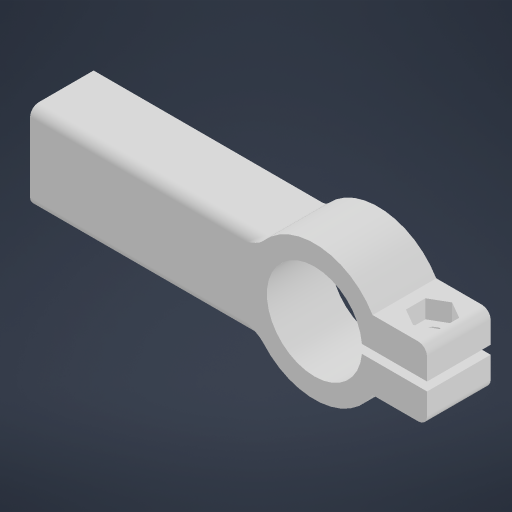
# Autodesk Inventor part: Clasp
Saved by Autodesk Inventor 2024.1 (Build 281209000, 209)
## iProperties
Created: 2023-09-06
Part Number: Clasp
Material: Generic
Document SubType Name: Modeling
Designer: User
Density: 1 g/cm^3
Appearance: Default
Author: User
Autodesk Inventor part; units mm, degrees
ref_plane "YZ Plane" through (0, 0, 0) normal (1, 0, 0) x (0, 1, 0)
ref_plane "XZ Plane" through (0, 0, 0) normal (0, 1, 0) x (-1, 0, 0)
ref_plane "XY Plane" through (0, 0, 0) normal (0, 0, 1) x (1, 0, 0)
sketch "Sketch1" plane through (0, 0, 0) normal (0, 0, 1) x (1, 0, 0)
  circle A0 centre (0, 0) radius 11
  circle A1 centre (0, 0) radius 15.6205
  line L0 (26, 8) -> (11, 8)
  line L1 (11, 8) -> (11, -8)
  line L2 (11, -8) -> (26, -8)
  line L3 (26, -8) -> (26, 8)
  line L4 (-65.7, 10) -> (-12, 10)
  line L5 (-12, 10) -> (-12, -10)
  line L6 (-12, -10) -> (-65.7, -10)
  line L7 (-65.7, -10) -> (-65.7, 10)
  point P0 (13.4164, 8)
  point P1 (13.4164, -8)
  point P2 (-12, -10)
  point P3 (-12, 10)
  point P4 (-12, 0)
  dimension "d0" = 22
  dimension "d1" = 31.241
  dimension "d10" = 15
  dimension "d11" = 16
  dimension "d45" = 53.7
  dimension "d46" = 20
  constraints: 16 end point, 4 parallel, 2 centre point, 2 coincident, 2 horizontal, 2 perpendicular, 1 midpoint, 2 other
  measures "d0" diameter of A0
  measures "d1" diameter of A1
  measures "d10" distance of L2.end L1.end
  measures "d11" distance of L1.end L0.end
  measures "d45" distance of L5.end L6.end
  measures "d46" distance of L4.end L5.end
extrude "Extrusion1" add sketch "Sketch1" along normal blind 14.7
sketch "Sketch2" plane through (0, 0, 14.7) normal (0, 0, 1) x (1, 0, 0)
  circle A0 centre (0, 0) radius 11 projected
  line L0 (26, -8) -> (26, 8) projected
  line L1 (26, 0) -> (10.8, 0)
  line L2 (10.8, 0) -> (10.8, 1)
  line L3 (10.8, 1) -> (26, 1)
  line L4 (26, 1) -> (26, 0)
  line L5 (26, 0) -> (10.8, 0)
  line L6 (10.8, 0) -> (10.8, -1)
  line L7 (10.8, -1) -> (26, -1)
  line L8 (26, -1) -> (26, 0)
  point P0 (10.9545, 1)
  point P1 (10.9545, -1)
  dimension "d20" = 15.2
  dimension "d21" = 1
  dimension "d22" = 1
  constraints: 16 end point, 4 parallel, 2 horizontal, 2 perpendicular, 1 midpoint, 1 point on line
  measures "d20" distance of L2.end L3.end
  measures "d21" distance of L1.end L2.end
  measures "d22" distance of L6.end L5.end
extrude "Extrusion2" cut sketch "Sketch2" against normal blind 15 contours L1 L2 L3 A0 | L1 L0 L7 A0 | A0 L3 L0 L1 | A0 L7 L6 L1
sketch "Sketch3" plane through (13.4164, -8, 0) normal (0, -1, 0) x (1, 0, 0)
  line L0 (0, 0) -> (0, 14.7) projected
  line L1 (0, 0) -> (6.6555, 0)
  line L2 (6.6555, 0) -> (6.6555, 7.5)
  line L3 (6.6555, 7.5) -> (0, 7.5)
  line L4 (0, 7.5) -> (0, 0)
  point P0 (-13.4164, 0)
  dimension "d25" = 6.6555
  dimension "d26" = 7.5
  constraints: 8 end point, 2 parallel, 1 coincident, 1 horizontal, 1 perpendicular
  measures "d25" distance of L3.end L2.end
  measures "d26" distance of L2.end L1.end
hole "Hole1" at (20.0719, -8, 7.5) direction (0, 1, 0) diameter 4.5 depth 12.5 counterbore diameter 8.5 counterbore depth 3.5
sketch "Sketch4" plane through (13.4164, 8, 0) normal (0, 1, 0) x (1, 0, 0)
  line L0 (12.5836, 0) -> (0, 0) projected
  line L1 (0, 0) -> (6.6555, 0)
  line L2 (6.6555, 0) -> (6.6555, -7.5)
  line L3 (6.6555, -7.5) -> (0, -7.5)
  line L4 (0, -7.5) -> (0, 0)
  line L5 (6.6555, -7.5) -> (6.6555, -12)
  line L6 (6.6555, -7.5) -> (11.1555, -7.5) construction
  line L7 (6.6555, -12) -> (2.7584, -9.75)
  line L8 (2.7584, -9.75) -> (2.7584, -5.25)
  line L9 (2.7584, -5.25) -> (6.6555, -3)
  line L10 (6.6555, -3) -> (10.5526, -5.25)
  line L11 (10.5526, -5.25) -> (10.5526, -9.75)
  line L12 (10.5526, -9.75) -> (6.6555, -12)
  point P0 (-13.4164, 0)
  dimension "d51" = 6.6555
  dimension "d52" = 7.5
  dimension "d53" = 4.5
  dimension "d54" = 90
  constraints: 24 end point, 2 coincident, 2 horizontal, 2 parallel, 2 perpendicular, 1 vertical, 13 other
  measures "d51" distance of L2.end L3.end
  measures "d52" distance of L1.end L2.end
  measures "d53" distance of L5.start L5.end
  measures "d54" angle of L5 L6
extrude "Extrusion3" cut sketch "Sketch4" against normal blind 4.2 contours L10 L11 L12 L5 L2 | L2 L3 L8 L9 | L5 L7 L8 L3
fillet "Fillet1" radius 2 2 edges at (-38.85, 10, 14.7) (-38.85, -10, 14.7)
fillet "Fillet2" radius 2 4 edges at (-12, -10, 6.35) (-12.4535, -9.4292, 14.0991) (-12, 10, 6.35) (-12.4535, 9.4292, 14.0991)
fillet "Fillet3" radius 2 2 edges at (26, -8, 7.35) (26, 8, 7.35)
body "Solid1"
